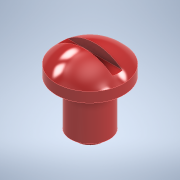
# Autodesk Inventor part: 1 Prisionero
Saved by Autodesk Inventor 2021 (Build 250183000, 183)
## iProperties
Created: 2020-10-13
Part Number: 1 Prisionero
Material: Steel
Document SubType Name: Modeling
Designer: valeg
Density: 7.85 g/cm^3
Appearance: Red
Author: valeg
Autodesk Inventor part; units mm, degrees
ref_plane "YZ Plane" through (0, 0, 0) normal (1, 0, 0) x (0, 1, 0)
ref_plane "XZ Plane" through (0, 0, 0) normal (0, 1, 0) x (-1, 0, 0)
ref_plane "XY Plane" through (0, 0, 0) normal (0, 0, 1) x (1, 0, 0)
sketch "Sketch1" plane through (0, 0, 0) normal (0, 1, 0) x (-1, 0, 0)
  circle A0 centre (0, 0) radius 5
  dimension "d0" = 10
  constraints: 1 centre point, 1 coincident
  measures "d0" diameter of A0
extrude "Extrusion1" add sketch "Sketch1" against normal blind 1.5
sketch "Sketch2" plane through (0, -1.5, 0) normal (0, -1, 0) x (1, 0, 0)
  circle A0 centre (0, 0) radius 2.875
  dimension "d3" = 5.75
  constraints: 1 centre point, 1 coincident
  measures "d3" diameter of A0
extrude "Extrusion2" add sketch "Sketch2" along normal blind 6.75
sketch "Sketch3" plane through (0, -8.25, 0) normal (0, -1, 0) x (1, 0, 0)
  circle A0 centre (0, 0) radius 2
  dimension "d6" = 4
  constraints: 1 centre point, 1 coincident
  measures "d6" diameter of A0
extrude "Extrusion3" add sketch "Sketch3" along normal blind 0.75
sketch "Sketch4" plane through (0, 0, 0) normal (1, 0, 0) x (0, 1, 0)
  line L0 (0, -5) -> (0, 5) projected
  arc A0 (0, -5) -> (0, 5) centre (-4.1533, 0) ccw
  line L1 (0, 5) -> (-0.75, 5)
  line L2 (0, 5) -> (-1.5, 5) projected
  line L3 (0, -5) -> (-1.5, -5) projected
  line L4 (-0.75, -5) -> (0, -5)
  line L5 (-4.1533, 5) -> (-4.1533, -5) construction
  point P0 (0, 0)
  dimension "d9" = 6.5
  constraints: 6 end point, 2 midpoint, 2 point on circle, 2 point on line, 1 centre point, 1 parallel, 1 perpendicular
  measures "d9" radius of A0
revolve "Revolution1" add sketch "Sketch4" angle 101 mid plane about axis through (0, -4.1533, 5) along (0, 0, -1)
sketch "Sketch5" plane through (0, 0, 0) normal (0, 1, 0) x (-1, 0, 0)
  circle A0 centre (0, 0) radius 5
  circle A1 centre (0, 0) radius 8.973
  constraints: 2 centre point, 2 coincident
extrude "Extrusion4" cut sketch "Sketch5" against normal mid plane 100
sketch "Sketch6" plane through (0, 0, 0) normal (1, 0, 0) x (0, 1, 0)
  line L0 (-8.25, 2.875) -> (-8.25, -2.875) projected
  line L1 (0.85, 0.75) -> (5.85, 0.75)
  line L2 (5.85, 0.75) -> (5.85, -0.75)
  line L3 (5.85, -0.75) -> (0.85, -0.75)
  line L4 (0.85, -0.75) -> (0.85, 0.75)
  point P0 (0, 0)
  dimension "d14" = 1.5
  dimension "d15" = 5
  constraints: 8 end point, 2 parallel, 1 horizontal, 1 perpendicular
  measures "d14" distance of L1.end L2.end
  measures "d15" distance of L2.end L3.end
extrude "Extrusion5" cut sketch "Sketch6" against normal mid plane 10
body "Solid1"
